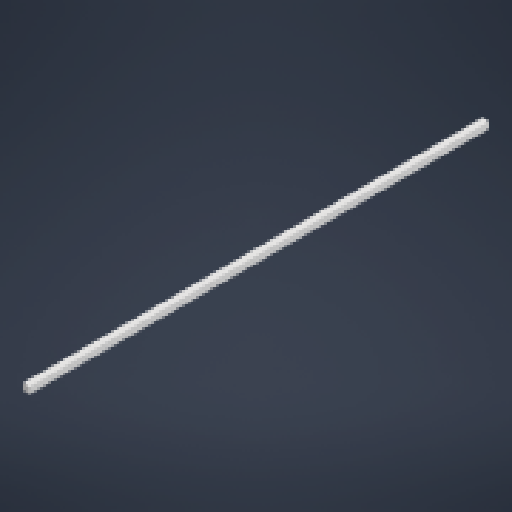
# Autodesk Inventor part: track
Saved by Autodesk Inventor 2023 (Build 270158000, 158)
## iProperties
Created: 2023-01-24
Part Number: track
Material: Generic
Document SubType Name: Modeling
Designer: Blank Slate
Density: 1 g/cm^3
Appearance: Default
Author: Blank Slate
Autodesk Inventor part; units mm, degrees
ref_plane "YZ Plane" through (0, 0, 0) normal (1, 0, 0) x (0, 1, 0)
ref_plane "XZ Plane" through (0, 0, 0) normal (0, 1, 0) x (-1, 0, 0)
ref_plane "XY Plane" through (0, 0, 0) normal (0, 0, 1) x (1, 0, 0)
sketch "Sketch1" plane through (0, 0, 0) normal (0, 1, 0) x (-1, 0, 0)
  line L0 (0, 0) -> (-152.4, 0)
  line L1 (-152.4, 0) -> (-152.4, -50.8)
  line L2 (-152.4, -50.8) -> (0, -50.8)
  line L3 (0, -50.8) -> (0, 0)
  line L4 (0, -25.4) -> (-152.4, -25.4) construction
  line L5 (0, -25.4) -> (-38.1, -25.4)
  line L6 (-152.4, -25.4) -> (-114.3, -25.4)
  circle A0 centre (-38.1, -25.4) radius 2.3813
  circle A1 centre (-114.3, -25.4) radius 2.3812
  dimension "d0" = 152.4
  dimension "d1" = 50.8
  dimension "d4" = 38.1
  dimension "d5" = 38.1
  dimension "d6" = 4.7625
  dimension "d7" = 4.7625
  constraints: 14 end point, 2 centre point, 2 coincident, 2 midpoint, 2 parallel, 2 point on line, 1 horizontal, 1 perpendicular
  measures "d0" distance of L2.end L1.end
  measures "d1" distance of L1.end L0.end
  measures "d4" distance of L4.start L5.end
  measures "d5" distance of L4.end L6.end
  measures "d6" diameter of A0
  measures "d7" diameter of A1
extrude "Extrusion1" add sketch "Sketch1" along normal blind 11.938 contours A1 | A0 | L3 L2 L1 L0
sketch "Sketch3" plane through (0, 11.938, 0) normal (0, 1, 0) x (1, 0, 0)
  line L0 (0, 50.8) -> (0, 0) projected
  line L1 (0, 25.4) -> (152.4, 25.4)
  line L2 (152.4, 0) -> (152.4, 50.8) projected
  line L3 (0, 25.4) -> (38.1, 25.4)
  line L4 (152.4, 25.4) -> (114.3, 25.4)
  line L5 (152.4, 25.4) -> (190.5, 25.4) construction
  circle A0 centre (38.1, 25.4) radius 2.3812
  circle A1 centre (114.3, 25.4) radius 2.3812
  dimension "d19" = 38.1
  dimension "d20" = 38.1
  dimension "d21" = 180
  dimension "d22" = 4.7625
  dimension "d23" = 4.7625
  constraints: 8 end point, 2 centre point, 2 coincident, 2 horizontal, 2 midpoint, 1 collinear, 1 point on line
  measures "d19" distance of L1.start L3.end
  measures "d20" distance of L1.end L4.end
  measures "d21" angle of L4 L5
  measures "d22" diameter of A0
  measures "d23" diameter of A1
hole "Hole2" at (38.1, 11.938, -25.4) at (114.3, 11.938, -25.4) direction (0, -1, 0) diameter 4.7625 end through all
body "Solid1"
